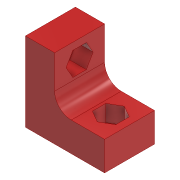
# Autodesk Inventor part: wheel box lid bracket
Saved by Autodesk Inventor 2020 (Build 240168000, 168)
## iProperties
Created: 2020-01-07
Part Number: wheel box lid bracket
Material: Generic
Document SubType Name: Modeling
Designer: ball
Density: 1 g/cm^3
Appearance: Default
Author: ball
Autodesk Inventor part; units mm, degrees
ref_plane "YZ Plane" through (0, 0, 0) normal (1, 0, 0) x (0, 1, 0)
ref_plane "XZ Plane" through (0, 0, 0) normal (0, 1, 0) x (-1, 0, 0)
ref_plane "XY Plane" through (0, 0, 0) normal (0, 0, 1) x (1, 0, 0)
sketch "Sketch1" plane through (0, 0, 0) normal (0, 1, 0) x (-1, 0, 0)
  line L0 (0, 0) -> (-12, 0)
  line L1 (-12, 0) -> (-12, -12)
  line L2 (-12, -12) -> (0, -12)
  line L3 (0, -12) -> (0, 0)
  dimension "d0" = 12
  dimension "d1" = 12
  constraints: 8 end point, 2 parallel, 1 horizontal, 1 perpendicular
  measures "d0" distance of L2.end L1.end
  measures "d1" distance of L1.end L0.end
extrude "Extrusion1" add sketch "Sketch1" along normal blind 7
sketch "Sketch2" plane through (0, 0, -12) normal (-1, 0, 0) x (0, 0, 1)
  line L0 (12, 0) -> (0, 0) projected
  line L1 (0, 0) -> (12, 0)
  line L2 (12, 0) -> (12, 19)
  line L3 (12, 19) -> (0, 19)
  line L4 (0, 19) -> (0, 0)
  dimension "d4" = 12
  dimension "d5" = 19
  constraints: 8 end point, 2 parallel, 1 horizontal, 1 perpendicular
  measures "d4" distance of L3.end L2.end
  measures "d5" distance of L2.end L1.end
extrude "Extrusion2" add sketch "Sketch2" along normal blind 7
sketch "Sketch3" plane through (0, 0, -12) normal (1, 0, 0) x (0, 0, -1)
  circle A0 centre (-6, 14.5) radius 3.25 construction
  line L0 (-12, 19) -> (0, 19) construction
  line L1 (-12, 7) -> (-12, 19) construction
  line L2 (-2.75, 14.5) -> (-4.375, 11.6854)
  line L3 (-4.375, 11.6854) -> (-7.625, 11.6854)
  line L4 (-7.625, 11.6854) -> (-9.25, 14.5)
  line L5 (-9.25, 14.5) -> (-7.625, 17.3146)
  line L6 (-7.625, 17.3146) -> (-4.375, 17.3146)
  line L7 (-4.375, 17.3146) -> (-2.75, 14.5)
  point P0 (-12, 0)
  dimension "d8" = 6.5
  dimension "d9" = 4.5
  dimension "d10" = 6
  constraints: 12 end point, 1 coincident, 1 horizontal alignment, 15 other
  measures "d9" distance from line of L0 point (-6, 14.5)
  measures "d10" distance from line of L1 point (-6, 14.5)
extrude "Extrusion3" cut sketch "Sketch3" against normal blind 4
sketch "Sketch4" plane through (0, 7, 0) normal (0, 1, 0) x (1, 0, 0)
  circle A0 centre (7.5, 6) radius 3.25 construction
  line L0 (12, 0) -> (12, 12) construction
  line L1 (12, 12) -> (0, 12) construction
  line L2 (0, 0) -> (12, 0) construction
  line L3 (7.5, 9.25) -> (10.3146, 7.625)
  line L4 (10.3146, 7.625) -> (10.3146, 4.375)
  line L5 (10.3146, 4.375) -> (7.5, 2.75)
  line L6 (7.5, 2.75) -> (4.6854, 4.375)
  line L7 (4.6854, 4.375) -> (4.6854, 7.625)
  line L8 (4.6854, 7.625) -> (7.5, 9.25)
  dimension "d13" = 6.5
  dimension "d14" = 4.5
  dimension "d15" = 6
  dimension "d16" = 12
  constraints: 12 end point, 1 coincident, 1 vertical alignment, 15 other
  measures "d14" distance from line of L0 point (7.5, 6)
  measures "d15" distance from line of L1 point (7.5, 6)
  measures "d16" distance between parallel lines of L1 L2
extrude "Extrusion4" cut sketch "Sketch4" against normal blind 4
fillet "Fillet1" radius 4 1 edges at (0, 7, -6)
sketch "Sketch7" plane through (0, 0, -12) normal (1, 0, 0) x (0, 0, -1)
  line L0 (-9.25, 14.5) -> (-7.625, 17.3146) construction
  line L1 (-4.375, 17.3146) -> (-2.75, 14.5) construction
  line L2 (-9.25, 14.5) -> (-2.75, 14.5) construction
  line L3 (-7.625, 17.3146) -> (-4.375, 17.3146) construction
  line L4 (-4.375, 11.6854) -> (-7.625, 11.6854) construction
  line L5 (-4.375, 17.3146) -> (-7.625, 11.6854) construction
  circle A0 centre (-6, 14.5) radius 1.7
  point P0 (-12, 0)
  dimension "d24" = 3.4
  constraints: 4 end point, 1 centre point, 1 horizontal, 1 midpoint
  measures "d24" diameter of A0
extrude "Extrusion7" cut sketch "Sketch7" against normal through all
sketch "Sketch8" plane through (0, 7, 0) normal (0, 1, 0) x (1, 0, 0)
  line L0 (7.5, 9.25) -> (10.3146, 7.625) construction
  line L1 (4.6854, 4.375) -> (4.6854, 7.625) construction
  line L2 (10.3146, 7.625) -> (4.6854, 4.375) construction
  line L3 (4.6854, 7.625) -> (7.5, 9.25) construction
  line L4 (10.3146, 7.625) -> (10.3146, 4.375) construction
  line L5 (4.6854, 7.625) -> (10.3146, 4.375) construction
  circle A0 centre (7.5, 6) radius 1.7
  point P0 (0, 0)
  dimension "d27" = 3.4
  constraints: 4 end point, 1 centre point, 1 midpoint
  measures "d27" diameter of A0
extrude "Extrusion8" cut sketch "Sketch8" against normal through all
equation "\"d15\" = 0.5 * d16"
body "Solid1"
